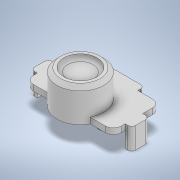
# Autodesk Inventor part: 로드셀 부품3
Saved by Autodesk Inventor 2021 (Build 250183000, 183)
## iProperties
Created: 2021-08-24
Part Number: 로드셀 부품3
Material: 일반
Document SubType Name: Modeling
Designer: Dongyoon
Density: 1 g/cm^3
Appearance: 기본값
Author: Dongyoon
Autodesk Inventor part; units mm, degrees
ref_plane "YZ Plane" through (0, 0, 0) normal (1, 0, 0) x (0, 1, 0)
ref_plane "XZ Plane" through (0, 0, 0) normal (0, 1, 0) x (-1, 0, 0)
sketch "스케치1" plane through (0, 0, 0) normal (0, 1, 0) x (-1, 0, 0)
  line L0 (9.25, -6) -> (-9.25, -6)
  line L1 (-11.25, -4) -> (-11.25, 4)
  line L2 (-9.25, 6) -> (9.25, 6)
  line L3 (11.25, 4) -> (11.25, -4)
  line L4 (11.25, -6) -> (-11.25, 6) construction
  line L5 (-11.25, -6) -> (11.25, 6) construction
  line L6 (5.5, -6) -> (5.5, -6.7)
  line L7 (4.5, -7.7) -> (-4.5, -7.7)
  line L8 (-5.5, -6.7) -> (-5.5, -6)
  line L9 (-11.25, -1.5) -> (-11.95, -1.5)
  line L10 (-12.95, -0.5) -> (-12.95, 2)
  line L11 (-11.95, 3) -> (-11.25, 3)
  line L12 (11.25, -1.5) -> (11.95, -1.5)
  line L13 (12.95, -0.5) -> (12.95, 2)
  line L14 (11.95, 3) -> (11.25, 3)
  arc A0 (9.25, -6) -> (11.25, -4) centre (9.25, -4) ccw
  arc A1 (-11.25, -4) -> (-9.25, -6) centre (-9.25, -4) ccw
  arc A2 (-9.25, 6) -> (-11.25, 4) centre (-9.25, 4) ccw
  arc A3 (11.25, 4) -> (9.25, 6) centre (9.25, 4) ccw
  arc A4 (12.95, 2) -> (11.95, 3) centre (11.95, 2) ccw
  arc A5 (11.95, -1.5) -> (12.95, -0.5) centre (11.95, -0.5) ccw
  arc A6 (4.5, -7.7) -> (5.5, -6.7) centre (4.5, -6.7) ccw
  arc A7 (-5.5, -6.7) -> (-4.5, -7.7) centre (-4.5, -6.7) ccw
  arc A8 (-12.95, -0.5) -> (-11.95, -1.5) centre (-11.95, -0.5) ccw
  arc A9 (-11.95, 3) -> (-12.95, 2) centre (-11.95, 2) ccw
  point P0 (0, 0)
  point P1 (5.5, -7.7)
  point P2 (-5.5, -7.7)
  point P3 (-12.95, 3)
  point P4 (12.95, -1.5)
  point P5 (12.95, 3)
  dimension "d0" = 22.5
  dimension "d1" = 12
  dimension "d2" = 11
  dimension "d3" = 5.5
  dimension "d4" = 1.7
  dimension "d5" = 9
  dimension "d6" = 1.7
  dimension "d7" = 1.7
  dimension "d8" = 4.5
  dimension "d9" = 2
  dimension "d10" = 1
  constraints: 30 end point, 28 point on line, 20 point on circle, 20 tangent, 10 centre point, 8 equal radius, 6 perpendicular, 2 horizontal, 2 midpoint, 2 parallel, 1 vertical
  measures "d0" distance of L4.start L5.start
  measures "d1" distance of L5.start L4.end
  measures "d2" distance of point (5.5, -7.7) point (-5.5, -7.7)
  measures "d3" distance from line of point (0, 0) L8
  measures "d4" distance of point (-5.5, -7.7) L8.end
  measures "d5" distance between parallel lines of L11 L0
  measures "d6" distance of point (-12.95, 3) L11.end
  measures "d7" distance of point (12.95, 3) L14.end
  measures "d8" distance between parallel lines of L9 L0
  measures "d9" radius of A0
  measures "d10" radius of A4
extrude "돌출1" add sketch "스케치1" against normal blind 1.5
sketch "스케치2" plane through (0, -1.5, 0) normal (0, -1, 0) x (1, 0, 0)
  line L0 (-11.25, 3) -> (-11.95, 3) projected
  line L1 (-11.25, -1.5) -> (-11.25, -4) projected
  line L2 (-11.25, 3) -> (-11.25, -1.5)
  line L3 (-11.25, -1.5) -> (-11.95, -1.5)
  line L4 (-12.95, -0.5) -> (-12.95, 2)
  line L5 (-11.95, 3) -> (-11.25, 3)
  line L6 (-11.25, 3) -> (-11.25, -1.5)
  line L7 (11.25, -4) -> (11.25, -1.5) projected
  line L8 (11.25, -1.5) -> (11.95, -1.5)
  line L9 (12.95, -0.5) -> (12.95, 2)
  line L10 (11.95, 3) -> (11.25, 3)
  line L11 (11.25, 3) -> (11.25, -1.5)
  line L12 (5.5, -6.7) -> (5.5, -6) projected
  line L13 (5.5, -6) -> (-5.5, -6)
  line L14 (-5.5, -6) -> (-5.5, -6.7)
  line L15 (-4.5, -7.7) -> (4.5, -7.7)
  line L16 (5.5, -6.7) -> (5.5, -6)
  arc A0 (-11.95, 3) -> (-12.95, 2) centre (-11.95, 2) ccw
  arc A1 (-12.95, -0.5) -> (-11.95, -1.5) centre (-11.95, -0.5) ccw
  arc A2 (12.95, 2) -> (11.95, 3) centre (11.95, 2) ccw
  arc A3 (11.95, -1.5) -> (12.95, -0.5) centre (11.95, -0.5) ccw
  arc A4 (4.5, -7.7) -> (5.5, -6.7) centre (4.5, -6.7) ccw
  arc A5 (-5.5, -6.7) -> (-4.5, -7.7) centre (-4.5, -6.7) ccw
  point P0 (0, 0)
  point P1 (12.95, 3)
  dimension "d13" = 1
  dimension "d14" = 9
  dimension "d15" = 1.7
  dimension "d16" = 1.7
  dimension "d17" = 4.5
  dimension "d18" = 1.7
  constraints: 26 end point, 12 point on circle, 12 tangent, 6 centre point, 6 parallel, 5 equal radius, 3 horizontal, 3 perpendicular, 3 point on line, 1 vertical
  measures "d13" radius of A0
  measures "d14" distance of L15.start L15.end
  measures "d15" distance between parallel lines of L15 L13
  measures "d16" distance between parallel lines of L11 L9
  measures "d17" distance of L10.end L7.end
  measures "d18" distance between parallel lines of L2 L4
extrude "돌출2" add sketch "스케치2" along normal blind 4
sketch "스케치3" plane through (0, -1.5, 0) normal (0, -1, 0) x (1, 0, 0)
  line L0 (-9.25, 6) -> (9.25, 6) projected
  line L1 (0, 6) -> (0, -6)
  line L2 (-5.5, -6) -> (5.5, -6) projected
  circle A0 centre (-5.95, 3.2) radius 1.25
  line L3 (-11.25, 4) -> (-11.25, 3) projected
  circle A1 centre (5.95, 3.2) radius 1.25
  point P0 (0, 0)
  dimension "d21" = 2.5
  dimension "d22" = 2.8
  dimension "d23" = 5.3
  constraints: 2 centre point, 2 end point, 2 midpoint, 1 symmetric about line, 1 other
  measures "d21" diameter of A0
  measures "d22" distance from line of L0 A0.centre
  measures "d23" distance from line of L3 A0.centre
extrude "돌출3" add sketch "스케치3" along normal blind 1.7
sketch "스케치4" plane through (0, 0, 0) normal (0, 1, 0) x (1, 0, 0)
  circle A0 centre (5.95, -3.2) radius 1.25 projected
  circle A1 centre (5.95, -3.2) radius 1.25
  circle A2 centre (-5.95, -3.2) radius 1.25 projected
  circle A3 centre (-5.95, -3.2) radius 1.25
  line L0 (5.95, -3.2) -> (-5.95, -3.2)
  circle A4 centre (0, -3.2) radius 6
  point P0 (0, 0)
  dimension "d26" = 12
  constraints: 3 centre point, 2 coincident, 2 end point, 1 horizontal, 1 midpoint
  measures "d26" diameter of A4
extrude "돌출4" add sketch "스케치4" along normal blind 7 contours A4 A0 | A0 L0 A2 A4 | A4 A2 L0 A0 | A2 A4 picked at (5.5714, -3.4284) picked at (-5.5569, -3.2)
sketch "스케치5" plane through (0, 0, 0) normal (0, -1, 0) x (1, 0, 0)
  arc A0 (5.3066, 6) -> (-5.3066, 6) centre (0, 3.2) ccw projected
  arc A1 (-5.3066, 6) -> (5.3066, 6) centre (0, 3.2) ccw projected
  arc A2 (5.3066, 6) -> (-5.3066, 6) centre (0, 3.2) ccw
  line L0 (-5.3066, 6) -> (5.3066, 6)
  line L1 (9.25, 6) -> (-9.25, 6) projected
  point P0 (0, 0)
  constraints: 2 end point, 2 point on circle, 2 point on line, 1 centre point, 1 coincident, 1 collinear
extrude "돌출5" add sketch "스케치5" along normal blind 1.5 contours L0 A0
ref_plane "작업 평면2" through (0, 0, 3.2) normal (0, 0, 1) x (1, 0, 0)
ref_plane "작업 평면1" through (0, 0, 9.2) normal (0, 0, 1) x (1, 0, 0)
sketch "스케치6" plane through (0, 0, 3.2) normal (0, 0, 1) x (1, 0, 0)
  line L0 (6, 7) -> (-6, 7) projected
  arc A0 (0, 11.25) -> (-4.25, 7) centre (0, 7) ccw
  line L1 (-4.25, 7) -> (0, 7)
  line L2 (-4.25, 7) -> (0, 7)
  line L3 (4.25, 7) -> (4.25, 7)
  line L4 (0, 6) -> (-3.25, 6)
  line L5 (-4.25, 7) -> (-4.25, 7)
  arc A1 (-4.25, 7) -> (-3.25, 6) centre (-3.25, 7) ccw
  line L6 (0, 7) -> (0, 1.0696)
  line L7 (0, 7) -> (0, 6)
  point P0 (0, 0)
  point P1 (4.25, 6)
  point P2 (-4.25, 6)
  point P3 (-4.25, 7)
  dimension "d32" = 8.5
  dimension "d35" = 8.5
  dimension "d36" = 1
  dimension "d37" = 1
  constraints: 14 end point, 7 point on line, 4 point on circle, 2 centre point, 2 parallel, 2 tangent, 2 vertical, 1 collinear, 1 horizontal, 1 midpoint, 1 perpendicular
  measures "d32" diameter of A0
  measures "d35" distance of point (4.25, 6) point (-4.25, 6)
  measures "d36" radius of A1
  measures "d37" distance between parallel lines of L0 L4
revolve "회전1" cut sketch "스케치6" angle 360 about axis through (0, 7, 3.2) along (0, -1, 0)
chamfer "모따기1" distance 1 angle 45 1 edges at (-6, 7, 3.2)
